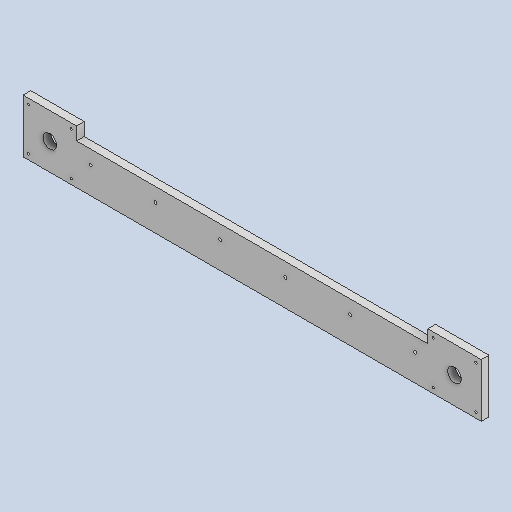
# Autodesk Inventor part: conveyor belt sideplank
Saved by Autodesk Inventor 2023 (Build 270158000, 158)
## iProperties
Created: 2022-06-04
Part Number: conveyor belt sideplank
Material: Generic
Document SubType Name: Modeling
Designer: prana_p9lsmih
Density: 1 g/cm^3
Appearance: Default
Author: prana_p9lsmih
Autodesk Inventor part; units mm, degrees
ref_plane "YZ Plane" through (0, 0, 0) normal (1, 0, 0) x (0, 1, 0)
ref_plane "XZ Plane" through (0, 0, 0) normal (0, 1, 0) x (-1, 0, 0)
ref_plane "XY Plane" through (0, 0, 0) normal (0, 0, 1) x (1, 0, 0)
sketch "Sketch1" plane through (0, 0, 0) normal (0, 0, 1) x (1, 0, 0)
  line L0 (-70, 0) -> (-70, 70)
  line L1 (-70, 70) -> (-140, 70)
  line L2 (-140, 70) -> (-140, 53)
  line L3 (-140, 53) -> (-600, 53)
  line L4 (-600, 53) -> (-600, 70)
  line L5 (-600, 70) -> (-670, 70)
  line L6 (-670, 70) -> (-670, 0)
  line L7 (-670, 0) -> (-70, 0)
  point P0 (0, 0)
  constraints: 16 end point, 4 perpendicular, 2 point on line, 1 horizontal
extrude "Extrusion1" add sketch "Sketch1" along normal blind 10
sketch "Sketch2" plane through (0, 0, 10) normal (0, 0, 1) x (1, 0, 0)
  line L0 (-70, 70) -> (-140, 70) projected
  line L1 (-70, 0) -> (-70, 70) projected
  line L2 (-600, 70) -> (-670, 70) projected
  line L3 (-670, 70) -> (-670, 0) projected
  point P0 (0, 0)
  point P1 (-105, 35)
  point P2 (-635, 35)
  dimension "d7" = 35
  dimension "d8" = 35
  dimension "d9" = 35
  dimension "d10" = 35
  measures "d7" distance from line of L0 point (-105, 35)
  measures "d8" distance from line of L1 point (-105, 35)
  measures "d9" distance from line of L2 point (-635, 35)
  measures "d10" distance from line of L3 point (-635, 35)
hole "Hole1" at (-105, 35, 10) at (-635, 35, 10) direction (0, 0, -1) diameter 18 end through all
sketch "Sketch3" plane through (0, 0, 10) normal (0, 0, 1) x (1, 0, 0)
  line L0 (-70, 70) -> (-140, 70) projected
  line L1 (-70, 0) -> (-70, 70) projected
  line L2 (-670, 0) -> (-70, 0) projected
  line L3 (-140, 70) -> (-140, 53) projected
  point P0 (0, 0)
  point P1 (-77, 63)
  point P2 (-77, 7)
  point P3 (-133, 63)
  point P4 (7, -7)
  dimension "d18" = 7
  dimension "d19" = 7
  dimension "d20" = 7
  dimension "d21" = 7
  dimension "d22" = 7
  dimension "d23" = 7
  dimension "d24" = 7
  measures "d18" distance from line of L0 point (-77, 63)
  measures "d19" distance from line of L1 point (-77, 63)
  measures "d20" distance from line of L2 point (-77, 7)
  measures "d21" distance from line of L1 point (-77, 7)
  measures "d22" distance from line of L0 point (-133, 63)
  measures "d23" distance from line of L3 point (-133, 63)
  measures "d24" distance from line of L2 point (7, -7)
hole "Hole2" at (-77, 63, 10) at (-77, 7, 10) at (-133, 63, 10) at (7, -7, 10) direction (0, 0, -1) diameter 3 end through all
sketch "Sketch4" plane through (0, 0, 10) normal (0, 0, 1) x (1, 0, 0)
  line L0 (-670, 0) -> (-70, 0) projected
  line L1 (-70, 0) -> (-70, 70) projected
  point P0 (0, 0)
  point P1 (-133, 7)
  dimension "d32" = 7
  dimension "d33" = 63
  measures "d32" distance from line of L0 point (-133, 7)
  measures "d33" distance from line of L1 point (-133, 7)
hole "Hole3" at (-133, 7, 10) direction (0, 0, -1) diameter 3 end through all
sketch "Sketch5" plane through (0, 0, 10) normal (0, 0, 1) x (1, 0, 0)
  line L0 (-600, 70) -> (-670, 70) projected
  line L1 (-670, 70) -> (-670, 0) projected
  line L2 (-670, 0) -> (-70, 0) projected
  line L3 (-600, 53) -> (-600, 70) projected
  point P0 (0, 0)
  point P1 (-663, 63)
  point P2 (-663, 7)
  point P3 (-607, 63)
  point P4 (-607, 7)
  dimension "d41" = 7
  dimension "d42" = 7
  dimension "d43" = 7
  dimension "d44" = 7
  dimension "d45" = 7
  dimension "d46" = 7
  dimension "d47" = 7
  dimension "d48" = 63
  measures "d41" distance from line of L0 point (-663, 63)
  measures "d42" distance from line of L1 point (-663, 63)
  measures "d43" distance from line of L2 point (-663, 7)
  measures "d44" distance from line of L1 point (-663, 7)
  measures "d45" distance from line of L0 point (-607, 63)
  measures "d46" distance from line of L3 point (-607, 63)
  measures "d47" distance from line of L2 point (-607, 7)
  measures "d48" distance from line of L1 point (-607, 7)
hole "Hole4" at (-663, 63, 10) at (-663, 7, 10) at (-607, 63, 10) at (-607, 7, 10) direction (0, 0, -1) diameter 3 end through all
sketch "Sketch6" plane through (0, 0, 10) normal (0, 0, 1) x (1, 0, 0)
  line L0 (-140, 53) -> (-600, 53) projected
  point P0 (0, 0)
  point P1 (-581.6285, 35)
  point P2 (-142, 53)
  point P3 (-598, 53)
  dimension "d63" = 18
  measures "d63" distance from line of L0 point (-581.628, 35)
hole "Hole5" at (-581.6285, 35, 10) direction (0, 0, -1) diameter 4 end through all
pattern_linear "Rectangular Pattern1" count 6 spacing 85 along (1, 0, 0) of "Hole5"
sketch "Sketch10" plane through (-670, 0, 0) normal (-1, 0, 0) x (0, 0, 1)
  line L0 (10, 70) -> (10, 0) projected
  line L1 (0, 0) -> (10, 0) projected
  point P0 (5, 35)
  dimension "d100" = 5
  dimension "d101" = 35
  measures "d100" distance from line of L0 point (5, 35)
  measures "d101" distance from line of L1 point (5, 35)
hole "Hole9" at (-670, 35, 5) direction (1, 0, 0) diameter 2 depth 10 tip angle 118
body "Solid1"
